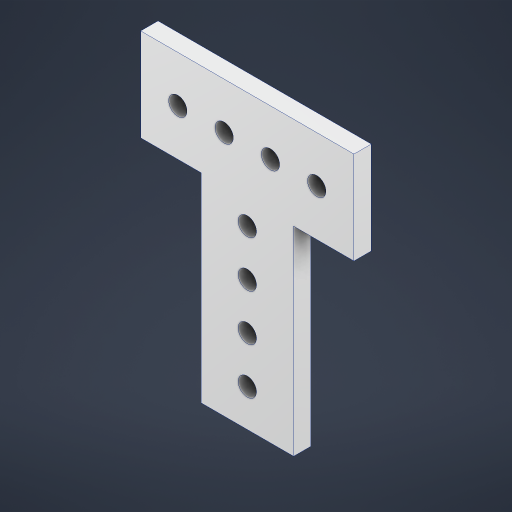
# Autodesk Inventor part: DVBS_006_T-bracket1
Saved by Autodesk Inventor 2024 (Build 280153000, 153)
## iProperties
Created: 2024-07-27
Part Number: DVBS_006_T-bracket1
Material: Aluminum 6061
Document SubType Name: Modeling
Designer: sarav
Density: 2.7 g/cm^3
Appearance: Aluminum - Flat
Author: sarav
Autodesk Inventor part; units mm, degrees
ref_plane "YZ Plane" through (0, 0, 0) normal (1, 0, 0) x (0, 1, 0)
ref_plane "XZ Plane" through (0, 0, 0) normal (0, 1, 0) x (-1, 0, 0)
ref_plane "XY Plane" through (0, 0, 0) normal (0, 0, 1) x (1, 0, 0)
sketch "Sketch1" plane through (0, 0, 0) normal (0, 0, 1) x (1, 0, 0)
  line L0 (0, 0) -> (25.4, 0)
  line L1 (25.4, 0) -> (25.4, 54.6608)
  line L2 (0, 54.6608) -> (0, 0)
  line L3 (0, 54.6608) -> (-16.5481, 54.6608)
  line L4 (-16.5481, 54.6608) -> (-16.5481, 80.0608)
  line L5 (-16.5481, 80.0608) -> (41.9481, 80.0608)
  line L6 (41.9481, 80.0608) -> (41.9481, 54.6608)
  line L7 (41.9481, 54.6608) -> (25.4, 54.6608)
  dimension "d0" = 25.4
  dimension "d1" = 54.6608
  dimension "d2" = 16.5481
  dimension "d3" = 25.4
  dimension "d4" = 58.4962
  dimension "d5" = 25.4
  dimension "d6" = 16.5481
  constraints: 16 end point, 4 perpendicular, 2 horizontal, 1 parallel, 1 point on line
  measures "d0" distance of L2.start L1.end
  measures "d1" distance of L1.end L0.end
  measures "d2" distance of L2.start L3.end
  measures "d3" distance of L3.end L4.end
  measures "d4" distance of L4.end L5.end
  measures "d5" distance of L5.end L6.end
  measures "d6" distance of L6.end L1.end
extrude "Extrusion1" add sketch "Sketch1" along normal blind 4.7625
sketch "Sketch2" plane through (0, 0, 4.7625) normal (0, 0, 1) x (1, 0, 0)
  line L0 (0, 0) -> (25.4, 0) projected
  line L1 (25.4, 0) -> (25.4, 54.6608) projected
  line L2 (25.4, 54.6608) -> (41.9481, 54.6608) projected
  line L3 (41.9481, 54.6608) -> (41.9481, 80.0608) projected
  line L4 (41.9481, 80.0608) -> (-16.5481, 80.0608) projected
  line L5 (-16.5481, 80.0608) -> (-16.5481, 54.6608) projected
  line L6 (-16.5481, 54.6608) -> (0, 54.6608) projected
  line L7 (0, 54.6608) -> (0, 0) projected
  circle A0 centre (-6.35, 67.3608) radius 2.5019
  circle A1 centre (6.35, 67.3608) radius 2.5019
  circle A2 centre (19.05, 67.3608) radius 2.5019
  circle A3 centre (31.75, 67.3608) radius 2.5019
  line L8 (34.2519, 67.3608) -> (41.9481, 67.3608)
  line L9 (0, 54.6608) -> (25.4, 54.6608)
  circle A4 centre (12.7, 48.2981) radius 2.5019
  circle A5 centre (12.7, 35.5981) radius 2.5019
  circle A6 centre (12.7, 22.8981) radius 2.5019
  circle A7 centre (12.7, 10.1981) radius 2.5019
  line L10 (12.7, 54.6608) -> (12.7, 50.8)
  line L11 (25.4, 0) -> (25.4, 54.6608) projected
  line L12 (12.7, 45.7962) -> (12.7, 38.1)
  line L13 (12.7, 33.0962) -> (12.7, 25.4)
  line L14 (12.7, 20.3962) -> (12.7, 12.7)
  dimension "d12" = 5.0038
  dimension "d24" = 5.0038
  dimension "d9" = 5.0038
  dimension "d10" = 5.0038
  dimension "d11" = 5.0038
  dimension "d13" = 12.7
  dimension "d20" = 7.6962
  dimension "d21" = 5.0038
  dimension "d22" = 5.0038
  dimension "d23" = 5.0038
  dimension "d25" = 3.8608
  dimension "d26" = 7.6962
  dimension "d27" = 7.6962
  dimension "d28" = 7.6962
  constraints: 12 end point, 8 point on line, 6 centre point, 6 point on circle, 3 vertical, 2 midpoint, 1 horizontal, 1 horizontal alignment, 1 parallel, 1 vertical alignment, 7 other
  measures "d9" diameter of A0
  measures "d10" diameter of A1
  measures "d11" diameter of A2
  measures "d13" distance from line of L4 point (31.75, 67.361)
  measures "d20" distance of L8.start L8.end
  measures "d21" diameter of A4
  measures "d22" diameter of A5
  measures "d23" diameter of A6
  measures "d25" distance of L10.start L10.end
  measures "d26" distance of L12.start L12.end
  measures "d27" distance of L13.start L13.end
  measures "d28" distance of L14.start L14.end
extrude "Extrusion2" cut sketch "Sketch2" against normal through all contours A0 | A1 | A2 | A3 | A4 | A5 | A6 | A7
body "Solid1"
